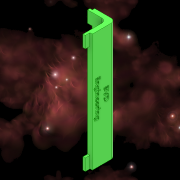
# Autodesk Inventor part: Klepje
Saved by Autodesk Inventor 2017 (Build 210142000, 142)
## iProperties
Created: 2016-12-19
Part Number: Klepje
Material: ABS Plastic
Document SubType Name: Modeling
Designer: bartv
Density: 1.06 g/cm^3
Appearance: Smooth - White
Author: bartv
Autodesk Inventor part; units mm, degrees
note: some values were not read from the file. Chosen so that the rebuilt part matches the saved one: direction of "Emboss1".
ref_plane "YZ Plane" through (0, 0, 0) normal (1, 0, 0) x (0, 1, 0)
ref_plane "XZ Plane" through (0, 0, 0) normal (0, 1, 0) x (-1, 0, 0)
ref_plane "XY Plane" through (0, 0, 0) normal (0, 0, 1) x (1, 0, 0)
sketch "Sketch1" plane through (0, 0, 0) normal (0, 0, 1) x (1, 0, 0)
  line L0 (0, 0) -> (-10, 0)
  line L1 (0, 0) -> (0, -10)
  line L2 (0, -10) -> (-2, -10)
  line L3 (-2, -10) -> (-2, -2)
  line L4 (-2, -2) -> (-10, -2)
  line L5 (-10, -2) -> (-10, 0)
  dimension "d0" = 10
  dimension "d1" = 10
  dimension "d2" = 2
  dimension "d3" = 8
  dimension "d4" = 2
  constraints: 12 end point, 2 perpendicular, 1 horizontal, 1 vertical
  measures "d0" distance of L0.start L0.end
  measures "d1" distance of L0.start L1.end
  measures "d2" distance of L1.end L2.end
  measures "d3" distance of L3.end L4.end
  measures "d4" distance between parallel lines of L0 L4
extrude "Extrusion1" add sketch "Sketch1" along normal blind 50.5
fillet "Fillet1" radius 2 2 edges at (0, 0, 25.25) (-2, -2, 25.25)
sketch "Sketch3" plane through (-2, -10, 0) normal (0, -1, 0) x (1, 0, 0)
  line L0 (0, 0) -> (1, 0)
  line L1 (1, 0) -> (1, 5)
  line L2 (1, 5) -> (0, 5)
  line L3 (0, 5) -> (0, 0)
  line L4 (2, 0) -> (2, 50.5) projected
  line L5 (0, 50.5) -> (2, 50.5) projected
  line L6 (0, 0) -> (0, 50.5) projected
  line L7 (0, 0) -> (0, 50.5) projected
  line L8 (0, 0) -> (2, 0) projected
  line L9 (2, 0) -> (2, 50.5) projected
  line L10 (0, 45.5) -> (1, 45.5)
  line L11 (1, 45.5) -> (1, 50.5)
  line L12 (1, 50.5) -> (0, 50.5)
  line L13 (0, 50.5) -> (0, 45.5)
  line L14 (2, 5) -> (0, 5) projected
  line L15 (0, 50.5) -> (2, 50.5) projected
  line L16 (0, 0) -> (2, 0) projected
  dimension "d13" = 1
  dimension "d14" = 1
  dimension "d15" = 5
  constraints: 16 end point, 4 parallel, 2 horizontal, 2 perpendicular, 1 collinear, 1 midpoint
  measures "d13" distance between parallel lines of L9 L1
  measures "d14" distance between parallel lines of L3 L1
  measures "d15" distance between parallel lines of L2 L0
extrude "Extrusion3" add sketch "Sketch3" along normal blind 2 contours L3 L2 L1 L0 | L6 L5 L11 L10
sketch "Sketch4" plane through (-10, 0, 50.5) normal (0, 1, 0) x (1, 0, 0)
  line L0 (8, 50.5) -> (8, 0) projected
  line L1 (8, 50.5) -> (0, 50.5) projected
  line L2 (0, 50.5) -> (0, 0) projected
  line L3 (8, 0) -> (0, 0) projected
  line L4 (0, 0) -> (1, 0)
  line L5 (1, 0) -> (1, 5)
  line L6 (1, 5) -> (0, 5)
  line L7 (0, 5) -> (0, 0)
  line L8 (0, 50.5) -> (1, 50.5)
  line L9 (1, 50.5) -> (1, 45.5)
  line L10 (1, 45.5) -> (0, 45.5)
  line L11 (0, 45.5) -> (0, 50.5)
  point P0 (10, 50.5)
  dimension "d18" = 5
  dimension "d19" = 1
  dimension "d20" = 5
  constraints: 16 end point, 4 parallel, 2 horizontal, 2 perpendicular, 1 point on line
  measures "d18" distance between parallel lines of L10 L1
  measures "d19" distance between parallel lines of L2 L9
  measures "d20" distance between parallel lines of L3 L6
extrude "Extrusion4" cut sketch "Sketch4" against normal blind 1 contours L9 L10 L2 L1 | L3 L2 L6 L5
sketch "Sketch5" plane through (-2, 0, 50.5) normal (0, 1, 0) x (1, 0, 0)
  line L0 (-7, 50.5) -> (-7, 45.5) projected
  line L1 (-7, 45.5) -> (-8, 45.5) projected
  line L2 (-8, 45.5) -> (-8, 5) projected
  line L3 (-8, 5) -> (-7, 5) projected
  line L4 (-7, 5) -> (-7, 0) projected
  line L5 (0, 0) -> (-7, 0) projected
  line L6 (0, 50.5) -> (0, 0) projected
  line L7 (0, 50.5) -> (-7, 50.5) projected
  line L8 (-8, 5) -> (-6, 5)
  line L9 (-6, 5) -> (-6, 45.5)
  line L10 (-6, 45.5) -> (-8, 45.5)
  line L11 (-8, 5) -> (-8, 45.5)
  point P0 (2, 50.5)
  dimension "d23" = 6
  constraints: 8 end point, 3 perpendicular, 1 horizontal
  measures "d23" distance between parallel lines of L6 L9
extrude "Extrusion5" cut sketch "Sketch5" against normal blind 2 contours L10 L9 L8 L3 L2 L1
sketch "Sketch6" plane through (0, -10, 50.5) normal (1, 0, 0) x (0, 0, -1)
  line L0 (13.101, 6.9901) -> (37.0866, 6.9901) construction
  line L1 (37.0866, 6.9901) -> (37.0866, 4.0966) construction
  line L2 (37.0866, 4.0966) -> (13.101, 4.0966) construction
  line L3 (13.101, 4.0966) -> (13.101, 6.9901) construction
  line L4 (0, 0) -> (0, 8) projected
  line L5 (0, 8) -> (50.5, 8) projected
  line L6 (22.4015, 4.9901) -> (22.4015, 6.9901)
  line L7 (22.4015, 6.9901) -> (23.1295, 6.9901)
  spline S0 degree 2 poles (23.1295, 6.9901) (23.4649, 6.9901) (23.8253, 6.7439) (23.8253, 6.5209) knots 0 0 0 1 2 2 2
  spline S1 degree 2 poles (23.8253, 6.5209) (23.8253, 6.3603) (23.6058, 6.1177) (23.4345, 6.0695) knots 0 0 0 1 2 2 2
  line L8 (23.4345, 6.0695) -> (23.4345, 6.0641)
  spline S2 degree 2 poles (23.4345, 6.0641) (23.6486, 6.0374) (23.9038, 5.7751) (23.9038, 5.5878) knots 0 0 0 1 2 2 2
  spline S3 degree 2 poles (23.9038, 5.5878) (23.9038, 5.313) (23.5113, 4.9901) (23.1705, 4.9901) knots 0 0 0 1 2 2 2
  line L9 (23.1705, 4.9901) -> (22.4015, 4.9901)
  line L10 (22.8529, 5.8501) -> (22.8529, 5.322)
  line L11 (22.8529, 5.322) -> (23.0973, 5.322)
  spline S4 degree 2 poles (23.0973, 5.322) (23.2526, 5.322) (23.4292, 5.4665) (23.4292, 5.5931) knots 0 0 0 1 2 2 2
  spline S5 degree 2 poles (23.4292, 5.5931) (23.4292, 5.7127) (23.2561, 5.8501) (23.0991, 5.8501) knots 0 0 0 1 2 2 2
  line L12 (23.0991, 5.8501) -> (22.8529, 5.8501)
  line L13 (22.8529, 6.6583) -> (22.8529, 6.1837)
  line L14 (22.8529, 6.1837) -> (23.051, 6.1837)
  spline S6 degree 2 poles (23.051, 6.1837) (23.1901, 6.1837) (23.3507, 6.3193) (23.3507, 6.437) knots 0 0 0 1 2 2 2
  spline S7 degree 2 poles (23.3507, 6.437) (23.3507, 6.6583) (23.0206, 6.6583) knots 0 0 0 1 1 1
  line L15 (23.0206, 6.6583) -> (22.8529, 6.6583)
  line L16 (25.8984, 6.9901) -> (25.208, 4.9901)
  line L17 (25.208, 4.9901) -> (24.6977, 4.9901)
  line L18 (24.6977, 4.9901) -> (24.018, 6.9901)
  line L19 (24.018, 6.9901) -> (24.5032, 6.9901)
  line L20 (24.5032, 6.9901) -> (24.9207, 5.5985)
  spline S8 degree 2 poles (24.9207, 5.5985) (24.9528, 5.4861) (24.96, 5.3987) knots 0 0 0 1 1 1
  line L21 (24.96, 5.3987) -> (24.9689, 5.3987)
  spline S9 degree 2 poles (24.9689, 5.3987) (24.9778, 5.4914) (25.0117, 5.6038) knots 0 0 0 1 1 1
  line L22 (25.0117, 5.6038) -> (25.4256, 6.9901)
  line L23 (25.4256, 6.9901) -> (25.8984, 6.9901)
  line L24 (26.1375, 4.9901) -> (26.1375, 6.9901)
  line L25 (26.1375, 6.9901) -> (26.8458, 6.9901)
  spline S10 degree 2 poles (26.8458, 6.9901) (27.9127, 6.9901) (27.9127, 6.016) knots 0 0 0 1 1 1
  spline S11 degree 2 poles (27.9127, 6.016) (27.9127, 5.5485) (27.3311, 4.9901) (26.8458, 4.9901) knots 0 0 0 1 2 2 2
  line L26 (26.8458, 4.9901) -> (26.1375, 4.9901)
  line L27 (26.5889, 6.6226) -> (26.5889, 5.3559)
  line L28 (26.5889, 5.3559) -> (26.8119, 5.3559)
  spline S12 degree 2 poles (26.8119, 5.3559) (27.1045, 5.3559) (27.4381, 5.7073) (27.4381, 6.0088) knots 0 0 0 1 2 2 2
  spline S13 degree 2 poles (27.4381, 6.0088) (27.4381, 6.2961) (27.108, 6.6226) (26.8083, 6.6226) knots 0 0 0 1 2 2 2
  line L29 (26.8083, 6.6226) -> (26.5889, 6.6226)
  line L30 (18.4765, 1.3707) -> (17.2758, 1.3707)
  line L31 (17.2758, 1.3707) -> (17.2758, 3.3707)
  line L32 (17.2758, 3.3707) -> (18.4301, 3.3707)
  line L33 (18.4301, 3.3707) -> (18.4301, 3.0031)
  line L34 (18.4301, 3.0031) -> (17.7271, 3.0031)
  line L35 (17.7271, 3.0031) -> (17.7271, 2.5589)
  line L36 (17.7271, 2.5589) -> (18.3801, 2.5589)
  line L37 (18.3801, 2.5589) -> (18.3801, 2.1931)
  line L38 (18.3801, 2.1931) -> (17.7271, 2.1931)
  line L39 (17.7271, 2.1931) -> (17.7271, 1.7364)
  line L40 (17.7271, 1.7364) -> (18.4765, 1.7364)
  line L41 (18.4765, 1.7364) -> (18.4765, 1.3707)
  line L42 (20.1321, 1.3707) -> (19.6932, 1.3707)
  line L43 (19.6932, 1.3707) -> (19.6932, 2.1646)
  spline S14 degree 2 poles (19.6932, 2.1646) (19.6932, 2.4964) (19.456, 2.4964) knots 0 0 0 1 1 1
  spline S15 degree 2 poles (19.456, 2.4964) (19.3418, 2.4964) (19.1937, 2.3198) (19.1937, 2.186) knots 0 0 0 1 2 2 2
  line L44 (19.1937, 2.186) -> (19.1937, 1.3707)
  line L45 (19.1937, 1.3707) -> (18.753, 1.3707)
  line L46 (18.753, 1.3707) -> (18.753, 2.7997)
  line L47 (18.753, 2.7997) -> (19.1937, 2.7997)
  line L48 (19.1937, 2.7997) -> (19.1937, 2.5732)
  line L49 (19.1937, 2.5732) -> (19.199, 2.5732)
  spline S16 degree 2 poles (19.199, 2.5732) (19.356, 2.8336) (19.6576, 2.8336) knots 0 0 0 1 1 1
  spline S17 degree 2 poles (19.6576, 2.8336) (20.1321, 2.8336) (20.1321, 2.2449) knots 0 0 0 1 1 1
  line L50 (20.1321, 2.2449) -> (20.1321, 1.3707)
  spline S18 degree 2 poles (21.8824, 1.533) (21.8824, 1.1369) (21.4221, 0.6998) (20.9849, 0.6998) knots 0 0 0 1 2 2 2
  spline S19 degree 2 poles (20.9849, 0.6998) (20.6959, 0.6998) (20.5282, 0.7819) knots 0 0 0 1 1 1
  line L51 (20.5282, 0.7819) -> (20.5282, 1.153)
  spline S20 degree 2 poles (20.5282, 1.153) (20.7477, 1.0245) (20.9725, 1.0245) knots 0 0 0 1 1 1
  spline S21 degree 2 poles (20.9725, 1.0245) (21.1955, 1.0245) (21.4417, 1.26) (21.4417, 1.4634) knots 0 0 0 1 2 2 2
  line L52 (21.4417, 1.4634) -> (21.4417, 1.5758)
  line L53 (21.4417, 1.5758) -> (21.4363, 1.5758)
  spline S22 degree 2 poles (21.4363, 1.5758) (21.2847, 1.335) (20.9903, 1.335) knots 0 0 0 1 1 1
  spline S23 degree 2 poles (20.9903, 1.335) (20.7173, 1.335) (20.3962, 1.7204) (20.3962, 2.0451) knots 0 0 0 1 2 2 2
  spline S24 degree 2 poles (20.3962, 2.0451) (20.3962, 2.4072) (20.753, 2.8336) (21.0456, 2.8336) knots 0 0 0 1 2 2 2
  spline S25 degree 2 poles (21.0456, 2.8336) (21.3061, 2.8336) (21.4363, 2.632) knots 0 0 0 1 1 1
  line L54 (21.4363, 2.632) -> (21.4417, 2.632)
  line L55 (21.4417, 2.632) -> (21.4417, 2.7997)
  line L56 (21.4417, 2.7997) -> (21.8824, 2.7997)
  line L57 (21.8824, 2.7997) -> (21.8824, 1.533)
  line L58 (21.447, 2.0576) -> (21.447, 2.17)
  spline S26 degree 2 poles (21.447, 2.17) (21.447, 2.3055) (21.2865, 2.4964) (21.158, 2.4964) knots 0 0 0 1 2 2 2
  spline S27 degree 2 poles (21.158, 2.4964) (21.0117, 2.4964) (20.844, 2.2681) (20.844, 2.0593) knots 0 0 0 1 2 2 2
  spline S28 degree 2 poles (20.844, 2.0593) (20.844, 1.8809) (21.0028, 1.674) (21.1419, 1.674) knots 0 0 0 1 2 2 2
  spline S29 degree 2 poles (21.1419, 1.674) (21.2775, 1.674) (21.447, 1.8845) (21.447, 2.0576) knots 0 0 0 1 2 2 2
  line L59 (22.6906, 1.3707) -> (22.2499, 1.3707)
  line L60 (22.2499, 1.3707) -> (22.2499, 2.7997)
  line L61 (22.2499, 2.7997) -> (22.6906, 2.7997)
  line L62 (22.6906, 2.7997) -> (22.6906, 1.3707)
  spline S30 degree 2 poles (22.4729, 3.0245) (22.3623, 3.0245) (22.2196, 3.1566) (22.2196, 3.2529) knots 0 0 0 1 2 2 2
  spline S31 degree 2 poles (22.2196, 3.2529) (22.2196, 3.3528) (22.3623, 3.4777) (22.4729, 3.4777) knots 0 0 0 1 2 2 2
  spline S32 degree 2 poles (22.4729, 3.4777) (22.5853, 3.4777) (22.7262, 3.3528) (22.7262, 3.2529) knots 0 0 0 1 2 2 2
  spline S33 degree 2 poles (22.7262, 3.2529) (22.7262, 3.153) (22.5853, 3.0245) (22.4729, 3.0245) knots 0 0 0 1 2 2 2
  line L63 (24.4408, 1.3707) -> (24.0019, 1.3707)
  line L64 (24.0019, 1.3707) -> (24.0019, 2.1646)
  spline S34 degree 2 poles (24.0019, 2.1646) (24.0019, 2.4964) (23.7646, 2.4964) knots 0 0 0 1 1 1
  spline S35 degree 2 poles (23.7646, 2.4964) (23.6504, 2.4964) (23.5023, 2.3198) (23.5023, 2.186) knots 0 0 0 1 2 2 2
  line L65 (23.5023, 2.186) -> (23.5023, 1.3707)
  line L66 (23.5023, 1.3707) -> (23.0617, 1.3707)
  line L67 (23.0617, 1.3707) -> (23.0617, 2.7997)
  line L68 (23.0617, 2.7997) -> (23.5023, 2.7997)
  line L69 (23.5023, 2.7997) -> (23.5023, 2.5732)
  line L70 (23.5023, 2.5732) -> (23.5077, 2.5732)
  spline S36 degree 2 poles (23.5077, 2.5732) (23.6647, 2.8336) (23.9662, 2.8336) knots 0 0 0 1 1 1
  spline S37 degree 2 poles (23.9662, 2.8336) (24.4408, 2.8336) (24.4408, 2.2449) knots 0 0 0 1 1 1
  line L71 (24.4408, 2.2449) -> (24.4408, 1.3707)
  line L72 (26.0733, 1.9594) -> (25.1419, 1.9594)
  spline S38 degree 2 poles (25.1419, 1.9594) (25.1634, 1.649) (25.5345, 1.649) knots 0 0 0 1 1 1
  spline S39 degree 2 poles (25.5345, 1.649) (25.77, 1.649) (25.9484, 1.7596) knots 0 0 0 1 1 1
  line L73 (25.9484, 1.7596) -> (25.9484, 1.442)
  spline S40 degree 2 poles (25.9484, 1.442) (25.7503, 1.335) (25.4328, 1.335) knots 0 0 0 1 1 1
  spline S41 degree 2 poles (25.4328, 1.335) (25.0866, 1.335) (24.7048, 1.7186) (24.7048, 2.0629) knots 0 0 0 1 2 2 2
  spline S42 degree 2 poles (24.7048, 2.0629) (24.7048, 2.4179) (25.1188, 2.8336) (25.4203, 2.8336) knots 0 0 0 1 2 2 2
  spline S43 degree 2 poles (25.4203, 2.8336) (25.7325, 2.8336) (26.0733, 2.4625) (26.0733, 2.145) knots 0 0 0 1 2 2 2
  line L74 (26.0733, 2.145) -> (26.0733, 1.9594)
  spline S44 degree 2 poles (25.6647, 2.2306) (25.6647, 2.5375) (25.4167, 2.5375) knots 0 0 0 1 1 1
  spline S45 degree 2 poles (25.4167, 2.5375) (25.3114, 2.5375) (25.1562, 2.3609) (25.1384, 2.2306) knots 0 0 0 1 2 2 2
  line L75 (25.1384, 2.2306) -> (25.6647, 2.2306)
  line L76 (27.6183, 1.9594) -> (26.687, 1.9594)
  spline S46 degree 2 poles (26.687, 1.9594) (26.7084, 1.649) (27.0795, 1.649) knots 0 0 0 1 1 1
  spline S47 degree 2 poles (27.0795, 1.649) (27.315, 1.649) (27.4934, 1.7596) knots 0 0 0 1 1 1
  line L77 (27.4934, 1.7596) -> (27.4934, 1.442)
  spline S48 degree 2 poles (27.4934, 1.442) (27.2954, 1.335) (26.9778, 1.335) knots 0 0 0 1 1 1
  spline S49 degree 2 poles (26.9778, 1.335) (26.6317, 1.335) (26.2499, 1.7186) (26.2499, 2.0629) knots 0 0 0 1 2 2 2
  spline S50 degree 2 poles (26.2499, 2.0629) (26.2499, 2.4179) (26.6638, 2.8336) (26.9653, 2.8336) knots 0 0 0 1 2 2 2
  spline S51 degree 2 poles (26.9653, 2.8336) (27.2775, 2.8336) (27.6183, 2.4625) (27.6183, 2.145) knots 0 0 0 1 2 2 2
  line L78 (27.6183, 2.145) -> (27.6183, 1.9594)
  spline S52 degree 2 poles (27.2097, 2.2306) (27.2097, 2.5375) (26.9618, 2.5375) knots 0 0 0 1 1 1
  spline S53 degree 2 poles (26.9618, 2.5375) (26.8565, 2.5375) (26.7013, 2.3609) (26.6834, 2.2306) knots 0 0 0 1 2 2 2
  line L79 (26.6834, 2.2306) -> (27.2097, 2.2306)
  spline S54 degree 2 poles (28.8119, 2.4019) (28.7334, 2.4447) (28.6263, 2.4447) knots 0 0 0 1 1 1
  spline S55 degree 2 poles (28.6263, 2.4447) (28.4836, 2.4447) (28.3213, 2.2342) (28.3213, 2.0522) knots 0 0 0 1 2 2 2
  line L80 (28.3213, 2.0522) -> (28.3213, 1.3707)
  line L81 (28.3213, 1.3707) -> (27.8806, 1.3707)
  line L82 (27.8806, 1.3707) -> (27.8806, 2.7997)
  line L83 (27.8806, 2.7997) -> (28.3213, 2.7997)
  line L84 (28.3213, 2.7997) -> (28.3213, 2.5339)
  line L85 (28.3213, 2.5339) -> (28.3266, 2.5339)
  spline S56 degree 2 poles (28.3266, 2.5339) (28.4319, 2.8247) (28.7031, 2.8247) knots 0 0 0 1 1 1
  spline S57 degree 2 poles (28.7031, 2.8247) (28.7726, 2.8247) (28.8119, 2.8069) knots 0 0 0 1 1 1
  line L86 (28.8119, 2.8069) -> (28.8119, 2.4019)
  line L87 (29.4577, 1.3707) -> (29.0171, 1.3707)
  line L88 (29.0171, 1.3707) -> (29.0171, 2.7997)
  line L89 (29.0171, 2.7997) -> (29.4577, 2.7997)
  line L90 (29.4577, 2.7997) -> (29.4577, 1.3707)
  spline S58 degree 2 poles (29.2401, 3.0245) (29.1295, 3.0245) (28.9867, 3.1566) (28.9867, 3.2529) knots 0 0 0 1 2 2 2
  spline S59 degree 2 poles (28.9867, 3.2529) (28.9867, 3.3528) (29.1295, 3.4777) (29.2401, 3.4777) knots 0 0 0 1 2 2 2
  spline S60 degree 2 poles (29.2401, 3.4777) (29.3525, 3.4777) (29.4934, 3.3528) (29.4934, 3.2529) knots 0 0 0 1 2 2 2
  spline S61 degree 2 poles (29.4934, 3.2529) (29.4934, 3.153) (29.3525, 3.0245) (29.2401, 3.0245) knots 0 0 0 1 2 2 2
  line L91 (31.208, 1.3707) -> (30.7691, 1.3707)
  line L92 (30.7691, 1.3707) -> (30.7691, 2.1646)
  spline S62 degree 2 poles (30.7691, 2.1646) (30.7691, 2.4964) (30.5318, 2.4964) knots 0 0 0 1 1 1
  spline S63 degree 2 poles (30.5318, 2.4964) (30.4176, 2.4964) (30.2695, 2.3198) (30.2695, 2.186) knots 0 0 0 1 2 2 2
  line L93 (30.2695, 2.186) -> (30.2695, 1.3707)
  line L94 (30.2695, 1.3707) -> (29.8288, 1.3707)
  line L95 (29.8288, 1.3707) -> (29.8288, 2.7997)
  line L96 (29.8288, 2.7997) -> (30.2695, 2.7997)
  line L97 (30.2695, 2.7997) -> (30.2695, 2.5732)
  line L98 (30.2695, 2.5732) -> (30.2749, 2.5732)
  spline S64 degree 2 poles (30.2749, 2.5732) (30.4319, 2.8336) (30.7334, 2.8336) knots 0 0 0 1 1 1
  spline S65 degree 2 poles (30.7334, 2.8336) (31.208, 2.8336) (31.208, 2.2449) knots 0 0 0 1 1 1
  line L99 (31.208, 2.2449) -> (31.208, 1.3707)
  spline S66 degree 2 poles (32.9582, 1.533) (32.9582, 1.1369) (32.4979, 0.6998) (32.0608, 0.6998) knots 0 0 0 1 2 2 2
  spline S67 degree 2 poles (32.0608, 0.6998) (31.7717, 0.6998) (31.604, 0.7819) knots 0 0 0 1 1 1
  line L100 (31.604, 0.7819) -> (31.604, 1.153)
  spline S68 degree 2 poles (31.604, 1.153) (31.8235, 1.0245) (32.0483, 1.0245) knots 0 0 0 1 1 1
  spline S69 degree 2 poles (32.0483, 1.0245) (32.2713, 1.0245) (32.5175, 1.26) (32.5175, 1.4634) knots 0 0 0 1 2 2 2
  line L101 (32.5175, 1.4634) -> (32.5175, 1.5758)
  line L102 (32.5175, 1.5758) -> (32.5122, 1.5758)
  spline S70 degree 2 poles (32.5122, 1.5758) (32.3605, 1.335) (32.0661, 1.335) knots 0 0 0 1 1 1
  spline S71 degree 2 poles (32.0661, 1.335) (31.7932, 1.335) (31.472, 1.7204) (31.472, 2.0451) knots 0 0 0 1 2 2 2
  spline S72 degree 2 poles (31.472, 2.0451) (31.472, 2.4072) (31.8288, 2.8336) (32.1214, 2.8336) knots 0 0 0 1 2 2 2
  spline S73 degree 2 poles (32.1214, 2.8336) (32.3819, 2.8336) (32.5122, 2.632) knots 0 0 0 1 1 1
  line L103 (32.5122, 2.632) -> (32.5175, 2.632)
  line L104 (32.5175, 2.632) -> (32.5175, 2.7997)
  line L105 (32.5175, 2.7997) -> (32.9582, 2.7997)
  line L106 (32.9582, 2.7997) -> (32.9582, 1.533)
  line L107 (32.5229, 2.0576) -> (32.5229, 2.17)
  spline S74 degree 2 poles (32.5229, 2.17) (32.5229, 2.3055) (32.3623, 2.4964) (32.2338, 2.4964) knots 0 0 0 1 2 2 2
  spline S75 degree 2 poles (32.2338, 2.4964) (32.0875, 2.4964) (31.9198, 2.2681) (31.9198, 2.0593) knots 0 0 0 1 2 2 2
  spline S76 degree 2 poles (31.9198, 2.0593) (31.9198, 1.8809) (32.0786, 1.674) (32.2178, 1.674) knots 0 0 0 1 2 2 2
  spline S77 degree 2 poles (32.2178, 1.674) (32.3534, 1.674) (32.5229, 1.8845) (32.5229, 2.0576) knots 0 0 0 1 2 2 2
  point P0 (50.5, 10)
  constraints: 2 other
emboss "Emboss1" sketch "Sketch6" operation cut depth 0.5 direction (-1, 0, 0)
body "Solid1"
